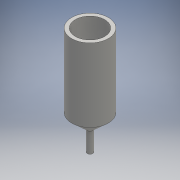
# Autodesk Inventor part: promo1
Saved by Autodesk Inventor 2016 (Build 200138000, 138)
## iProperties
Created: 2016-05-06
Part Number: promo1
Material: 一般
Document SubType Name: Modeling
Designer: 宏太
Density: 1 g/cm^3
Appearance: 既定
Author: 宏太
Autodesk Inventor part; units mm, degrees
ref_plane "YZ Plane" through (0, 0, 0) normal (1, 0, 0) x (0, 1, 0)
ref_plane "XZ Plane" through (0, 0, 0) normal (0, 1, 0) x (-1, 0, 0)
ref_plane "XY Plane" through (0, 0, 0) normal (0, 0, 1) x (1, 0, 0)
sketch "スケッチ1" plane through (0, 0, 0) normal (0, 1, 0) x (-1, 0, 0)
  line L0 (0, 0) -> (20, 0) construction
  line L1 (20, 0) -> (20, 80)
  line L2 (20, 80) -> (0, 80)
  line L3 (20, 0) -> (0, 0)
  line L4 (0, 80) -> (0, 0)
  dimension "d4" = 80
  dimension "d12" = 20
  constraints: 10 end point, 2 vertical, 1 collinear, 1 horizontal, 1 perpendicular
  measures "d4" distance of L0.end L1.end
  measures "d12" distance of L1.end L2.end
revolve "回転1" add sketch "スケッチ1" angle 360 about axis through (0, 0, 80) along (0, 0, -1)
shell "シェル1" thickness 4 removed faces 1 at (-3.567, 7.2992, 80)
sketch "スケッチ2" plane through (0, 0, 0) normal (0, 1, 0) x (-1, 0, 0)
  line L0 (-20, 0) -> (20, 0) projected
  line L1 (0, -17.2687) -> (0, 0)
  line L2 (0, 0) -> (20, 0)
  line L3 (0, -17.2687) -> (0, -37.2687)
  line L4 (0, -37.2687) -> (3, -37.2687)
  line L5 (3, -37.2687) -> (3, -15.5418)
  line L6 (20, 0) -> (3, -15.5418)
  dimension "d9" = 20
  dimension "d10" = 3
  constraints: 12 end point, 3 perpendicular, 1 collinear, 1 vertical
  measures "d9" distance of L1.start L3.end
  measures "d10" distance of L3.end L4.end
revolve "回転2" add sketch "スケッチ2" angle 360 about axis through (0, 0, -17.2687) along (0, 0, 1)
